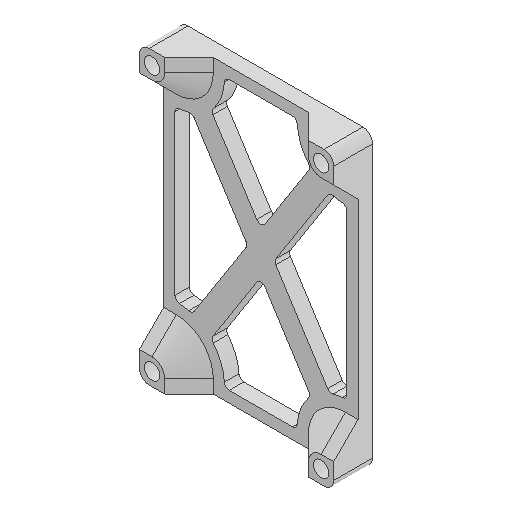
# Autodesk Inventor part: Test_PCB_Board_4x6
Saved by Autodesk Inventor 2026.2 (Build 302298000, 298)
## iProperties
Created: 2026-05-06
Part Number: Test_PCB_Board_4x6
Material: Generic
Document SubType Name: Modeling
Designer: pacoa
Density: 1 g/cm^3
Appearance: Default
Author: pacoa
Autodesk Inventor part; units mm, degrees
ref_plane "YZ Plane" through (0, 0, 0) normal (1, 0, 0) x (0, 1, 0)
ref_plane "XZ Plane" through (0, 0, 0) normal (0, 1, 0) x (-1, 0, 0)
ref_plane "XY Plane" through (0, 0, 0) normal (0, 0, 1) x (1, 0, 0)
sketch "Sketch1" plane through (0, 0, 0) normal (0, 1, 0) x (-1, 0, 0)
  line L0 (0, 0) -> (40, 0)
  line L1 (40, 0) -> (40, -60)
  line L2 (40, -60) -> (0, -60)
  line L3 (0, -60) -> (0, 0)
  circle A0 centre (2.6, -2.75) radius 1.27
  circle A1 centre (37.4, -2.75) radius 1.27
  circle A2 centre (37.4, -57.25) radius 1.27
  circle A3 centre (2.6, -57.25) radius 1.27
  dimension "d1" = 40
  dimension "d2" = 60
  dimension "d15" = 2.54
  dimension "d20" = 2.75
  dimension "d21" = 2.6
  dimension "d22" = 2.54
  dimension "d23" = 2.75
  dimension "d24" = 2.6
  dimension "d25" = 2.54
  dimension "d26" = 2.54
  dimension "d27" = 2.75
  dimension "d28" = 2.75
  dimension "d29" = 2.6
  dimension "d30" = 2.6
  constraints: 8 end point, 4 centre point, 2 parallel, 1 horizontal, 1 perpendicular
  measures "d1" distance of L1.end L2.end
  measures "d2" distance of L0.end L1.end
  measures "d15" diameter of A0
  measures "d20" distance from line of L0 A0.centre
  measures "d21" distance from line of L3 A0.centre
  measures "d22" diameter of A1
  measures "d23" distance from line of L0 A1.centre
  measures "d24" distance from line of L1 A1.centre
  measures "d25" diameter of A2
  measures "d26" diameter of A3
  measures "d27" distance from line of L2 A2.centre
  measures "d28" distance from line of L2 A3.centre
  measures "d29" distance from line of L3 A3.centre
  measures "d30" distance from line of L1 A2.centre
extrude "Extrusion1" add sketch "Sketch1" along normal blind 3 contours L0 L1 L2 L3 | A0 | A1 | A2 | A3
sketch "Sketch2" plane through (0, 0, 0) normal (0, -1, 0) x (1, 0, 0)
  line L0 (-40, 0) -> (0, 0) projected
  line L1 (0, -60) -> (-40, -60) projected
  arc A0 (-5.2, -2.75) -> (-2.6, -5.35) centre (-2.6, -2.75) ccw
  line L2 (0, 0) -> (0, -60) projected
  arc A1 (-2.6, -54.65) -> (-5.2, -57.25) centre (-2.6, -57.25) ccw
  arc A2 (-34.8, -57.25) -> (-37.4, -54.65) centre (-37.4, -57.25) ccw
  line L3 (-40, -60) -> (-40, 0) projected
  arc A3 (-37.4, -5.35) -> (-34.8, -2.75) centre (-37.4, -2.75) ccw
  line L4 (-34.8, -57.25) -> (-34.8, -60)
  line L5 (-34.8, -2.75) -> (-34.8, 0)
  line L6 (-5.2, -57.25) -> (-5.2, -60)
  line L7 (-5.2, -2.75) -> (-5.2, 0)
  line L8 (-37.4, -54.65) -> (-40, -54.65)
  line L9 (0, -5.35) -> (-2.6, -5.35)
  line L10 (-37.4, -5.35) -> (-40, -5.35)
  line L11 (-40, -54.65) -> (-37.4, -54.65)
  line L12 (-2.6, -54.65) -> (0, -54.65)
  constraints: 18 end point, 8 point on circle, 8 point on line, 4 centre point, 4 coincident, 4 tangent, 4 vertical, 3 horizontal
extrude "Extrusion2" add sketch "Sketch2" along normal blind 5 contours L0 L5 A3 L10 L3 | L0 L2 L9 A0 L7 | L8 A2 L4 L1 L3 | L2 L1 L6 A1 L12
sketch "Sketch4" plane through (0, -5, 0) normal (0, -1, 0) x (1, 0, 0)
  arc A0 (-2.6, -54.65) -> (-5.2, -57.25) centre (-2.6, -57.25) ccw projected
  arc A1 (-34.8, -57.25) -> (-37.4, -54.65) centre (-37.4, -57.25) ccw projected
  arc A2 (-5.2, -2.75) -> (-2.6, -5.35) centre (-2.6, -2.75) ccw projected
  arc A3 (-37.4, -5.35) -> (-34.8, -2.75) centre (-37.4, -2.75) ccw projected
  point P0 (0, 0)
  constraints: 4 coincident
hole "Hole2" at (-2.6, -5, -57.25) at (-37.4, -5, -57.25) at (-2.6, -5, -2.75) at (-37.4, -5, -2.75) direction (0, 1, 0) diameter 3.2 depth 4 tip angle 118
chamfer "Chamfer1" distance 5 angle 45 12 edges at (-1.3, 0, -54.65) (-4.4385, 0, -55.4115) (-5.2, 0, -58.625) (-35.5615, 0, -55.4115) (-34.8, 0, -58.625) (-38.7, 0, -54.65) (-35.5615, 0, -4.5885) (-38.7, 0, -5.35) (-34.8, 0, -1.375) (-1.3, 0, -5.35) (-4.4385, 0, -4.5885) (-5.2, 0, -1.375)
sketch "Sketch5" plane through (0, 0, 0) normal (0, -1, 0) x (1, 0, 0)
  line L0 (-10.2, 0) -> (-10.2, -2.75) projected
  line L1 (-29.8, 0) -> (-10.2, 0) projected
  line L2 (-29.8, -2.75) -> (-29.8, 0) projected
  arc A0 (-37.4, -10.35) -> (-29.8, -2.75) centre (-37.4, -2.75) ccw projected
  line L3 (-40, -10.35) -> (-37.4, -10.35) projected
  line L4 (-40, -49.65) -> (-40, -10.35) projected
  line L5 (-37.4, -49.65) -> (-40, -49.65) projected
  arc A1 (-29.8, -57.25) -> (-37.4, -49.65) centre (-37.4, -57.25) ccw projected
  line L6 (-29.8, -60) -> (-29.8, -57.25) projected
  line L7 (-10.2, -60) -> (-29.8, -60) projected
  line L8 (-10.2, -57.25) -> (-10.2, -60) projected
  arc A2 (-2.6, -49.65) -> (-10.2, -57.25) centre (-2.6, -57.25) ccw projected
  line L9 (0, -49.65) -> (-2.6, -49.65) projected
  line L10 (0, -10.35) -> (0, -49.65) projected
  line L11 (-2.6, -10.35) -> (0, -10.35) projected
  arc A3 (-10.2, -2.75) -> (-2.6, -10.35) centre (-2.6, -2.75) ccw projected
  line L12 (-12.5, -57.25) -> (-12.5, -57.7)
  line L13 (-13.4861, -57.7) -> (-26.5139, -57.7)
  line L14 (-27.5, -57.7) -> (-27.5, -57.25)
  line L15 (-37.4, -47.35) -> (-37.7, -47.35)
  line L16 (-37.7, -46.3725) -> (-37.7, -13.6275)
  line L17 (-37.7, -12.65) -> (-37.4, -12.65)
  line L18 (-27.5, -2.75) -> (-27.5, -2.3)
  line L19 (-26.5139, -2.3) -> (-13.4861, -2.3)
  line L20 (-12.5, -2.3) -> (-12.5, -2.75)
  line L21 (-2.6, -12.65) -> (-2.3, -12.65)
  line L22 (-2.3, -13.6275) -> (-2.3, -46.3725)
  line L23 (-2.3, -47.35) -> (-2.6, -47.35)
  line L24 (0, -60) -> (-40, -60) projected
  arc A4 (-5.2, -2.75) -> (-2.6, -5.35) centre (-2.6, -2.75) ccw projected
  circle A5 centre (-37.4, -2.75) radius 1.6 projected
  line L25 (-0.6615, -56.0122) -> (-2.3, -53.4461)
  line L26 (-4.5385, -58.4878) -> (-5.0416, -57.7)
  line L27 (-34.9584, -57.7) -> (-35.4615, -58.4878)
  line L28 (-37.7, -53.4461) -> (-39.3385, -56.0122)
  arc A6 (-3.2358, -47.3704) -> (-5.1517, -47.6845) centre (-2.6, -57.25) ccw
  arc A7 (-10.2041, -50.9106) -> (-12.4874, -56.7505) centre (-2.6, -57.25) ccw
  arc A8 (-27.5126, -56.7505) -> (-29.7959, -50.9106) centre (-37.4, -57.25) ccw
  arc A9 (-34.8483, -47.6845) -> (-36.7642, -47.3704) centre (-37.4, -57.25) ccw
  arc A10 (-36.7642, -12.6296) -> (-34.8483, -12.3155) centre (-37.4, -2.75) ccw
  arc A11 (-29.7959, -9.0894) -> (-27.5126, -3.2495) centre (-37.4, -2.75) ccw
  arc A12 (-12.4874, -3.2495) -> (-10.2041, -9.0894) centre (-2.6, -2.75) ccw
  arc A13 (-5.1517, -12.3155) -> (-3.2358, -12.6296) centre (-2.6, -2.75) ccw
  line L29 (-6.2523, -47.2565) -> (-16.9275, -30.5382)
  line L30 (-20.8428, -24.4063) -> (-29.8707, -10.2679)
  line L31 (-6.2523, -12.7435) -> (-16.9275, -29.4618)
  line L32 (-20.8428, -35.5937) -> (-29.8707, -49.7321)
  line L33 (-10.1293, -49.7321) -> (-19.1572, -35.5937)
  line L34 (-23.0725, -29.4618) -> (-33.7477, -12.7435)
  line L35 (-10.1293, -10.2679) -> (-19.1572, -24.4063)
  line L36 (-23.0725, -30.5382) -> (-33.7477, -47.2565)
  arc A14 (-3.2358, -47.3704) -> (-2.3, -46.3725) centre (-3.3, -46.3725) ccw
  arc A15 (-6.2523, -47.2565) -> (-5.1517, -47.6845) centre (-5.4095, -46.7183) ccw
  arc A16 (-10.2041, -50.9106) -> (-10.1293, -49.7321) centre (-10.9722, -50.2703) ccw
  arc A17 (-13.4861, -57.7) -> (-12.4874, -56.7505) centre (-13.4861, -56.7) ccw
  arc A18 (-27.5126, -56.7505) -> (-26.5139, -57.7) centre (-26.5139, -56.7) ccw
  arc A19 (-29.8707, -49.7321) -> (-29.7959, -50.9106) centre (-29.0278, -50.2703) ccw
  arc A20 (-34.8483, -47.6845) -> (-33.7477, -47.2565) centre (-34.5905, -46.7183) ccw
  arc A21 (-37.7, -46.3725) -> (-36.7642, -47.3704) centre (-36.7, -46.3725) ccw
  arc A22 (-36.7642, -12.6296) -> (-37.7, -13.6275) centre (-36.7, -13.6275) ccw
  arc A23 (-33.7477, -12.7435) -> (-34.8483, -12.3155) centre (-34.5905, -13.2817) ccw
  arc A24 (-23.0725, -30.5382) -> (-23.0725, -29.4618) centre (-23.9154, -30) ccw
  arc A25 (-19.1572, -35.5937) -> (-20.8428, -35.5937) centre (-20, -36.1318) ccw
  arc A26 (-16.9275, -29.4618) -> (-16.9275, -30.5382) centre (-16.0846, -30) ccw
  arc A27 (-20.8428, -24.4063) -> (-19.1572, -24.4063) centre (-20, -23.8682) ccw
  arc A28 (-5.1517, -12.3155) -> (-6.2523, -12.7435) centre (-5.4095, -13.2817) ccw
  arc A29 (-2.3, -13.6275) -> (-3.2358, -12.6296) centre (-3.3, -13.6275) ccw
  arc A30 (-10.1293, -10.2679) -> (-10.2041, -9.0894) centre (-10.9722, -9.7297) ccw
  arc A31 (-12.4874, -3.2495) -> (-13.4861, -2.3) centre (-13.4861, -3.3) ccw
  arc A32 (-26.5139, -2.3) -> (-27.5126, -3.2495) centre (-26.5139, -3.3) ccw
  arc A33 (-29.7959, -9.0894) -> (-29.8707, -10.2679) centre (-29.0278, -9.7297) ccw
  point P0 (0, 0)
  point P1 (-34.1564, -12.1035)
  point P2 (-30.2793, -9.6279)
  point P3 (-5.8436, -12.1035)
  point P4 (-9.7207, -9.6279)
  point P5 (-5.8436, -47.8965)
  point P6 (-9.7207, -50.3721)
  point P7 (-30.2793, -50.3721)
  point P8 (-34.1564, -47.8965)
  dimension "d57" = 1
  constraints: 72 point on circle, 48 end point, 40 tangent, 28 centre point, 20 point on line, 19 equal radius, 8 other
  measures "d57" radius of A14
extrude "Extrusion3" cut sketch "Sketch5" against normal through all contours L13 A18 A8 A19 L32 A25 L33 A16 A7 A17 | L16 A22 A10 A23 L34 A24 L36 A20 A9 A21 | L19 A31 A12 A30 L35 A27 L30 A33 A11 A32 | L22 A14 A6 A15 L29 A26 L31 A28 A13 A29
fillet "Fillet1" [suppressed]
fillet "Fillet2" radius 2 4 edges at (-40, -1, 0) (-40, -1, -60) (0, -1, -60) (0, -1, 0)
equation "\"d23\" = d20"
equation "\"d24\" = d21"
equation "\"d27\" = d23"
equation "\"d28\" = d20"
equation "\"d29\" = d21"
equation "\"d30\" = d21"
body "Solid1"
